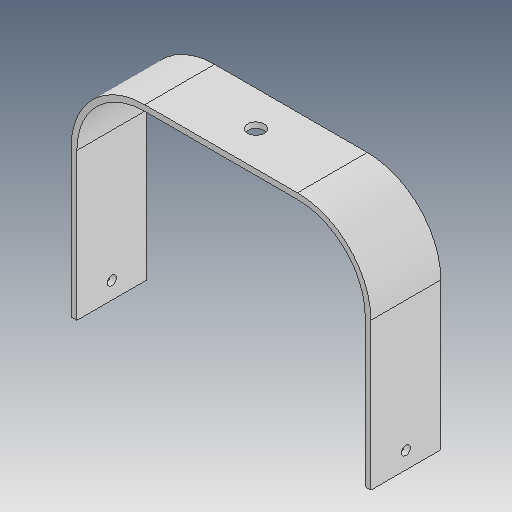
# Autodesk Inventor part: pulley_bracket
Saved by Autodesk Inventor 2025.2 (Build 292293000, 293)
## iProperties
Created: 2025-02-16
Part Number: pulley_bracket
Material: Generic
Document SubType Name: Modeling
Designer: email
Density: 1 g/cm^3
Appearance: Default
Author: email
Autodesk Inventor part; units mm, degrees
ref_plane "YZ Plane" through (0, 0, 0) normal (1, 0, 0) x (0, 1, 0)
ref_plane "XZ Plane" through (0, 0, 0) normal (0, 1, 0) x (-1, 0, 0)
ref_plane "XY Plane" through (0, 0, 0) normal (0, 0, 1) x (1, 0, 0)
sketch "Sketch1" plane through (0, 0, 0) normal (0, 0, 1) x (1, 0, 0)
  line L0 (0, 0) -> (0, 80)
  line L1 (163, 0) -> (163, 80)
  line L2 (0, 0) -> (3.1, 0)
  line L3 (3.1, 0) -> (3.1, 80)
  line L4 (163, 0) -> (159.9, 0)
  line L5 (159.9, 0) -> (159.9, 80)
  arc A0 (40, 116.9) -> (3.1, 80) centre (40, 80) ccw
  arc A1 (159.9, 80) -> (123, 116.9) centre (123, 80) ccw
  line L6 (40, 116.9) -> (123, 116.9)
  arc A2 (40, 120) -> (0, 80) centre (40, 80) ccw
  line L7 (40, 120) -> (123, 120)
  arc A3 (163, 80) -> (123, 120) centre (123, 80) ccw
  dimension "d0" = 163
  dimension "d1" = 80
  dimension "d2" = 3.1
  dimension "d3" = 3.1
  dimension "d4" = 3.1
  dimension "d5" = 120
  constraints: 16 end point, 8 point on circle, 6 tangent, 4 centre point, 4 horizontal, 2 concentric, 2 perpendicular, 2 vertical, 1 collinear, 1 parallel
  measures "d0" distance between parallel lines of L1 L0
  measures "d1" distance of L0.start L0.end
  measures "d2" distance between parallel lines of L0 L3
  measures "d3" distance between parallel lines of L1 L5
  measures "d4" distance between parallel lines of L7 L6
  measures "d5" distance between parallel lines of L7 L2
extrude "Extrusion1" add sketch "Sketch1" along normal blind 38
sketch "Sketch2" plane through (163, 0, 0) normal (1, 0, 0) x (0, 0, -1)
  circle A0 centre (-19, 9.25) radius 2.5
  line L0 (-38, 0) -> (-38, 80) projected
  line L1 (0, 0) -> (-38, 0) projected
  dimension "d8" = 5
  dimension "d9" = 19
  dimension "d10" = 9.25
  constraints: 1 centre point
  measures "d8" diameter of A0
  measures "d9" distance from line of L0 A0.centre
  measures "d10" distance from line of L1 A0.centre
extrude "Extrusion2" cut sketch "Sketch2" against normal through all
sketch "Sketch3" plane through (40, 120, 0) normal (0, 1, 0) x (1, 0, 0)
  circle A0 centre (41.5, -19) radius 4.5
  line L0 (-40, 0) -> (-40, -38) projected
  line L1 (83, 0) -> (0, 0) projected
  point P0 (-40, -19)
  dimension "d13" = 81.5
  dimension "d14" = 19
  dimension "d15" = 9
  constraints: 1 centre point, 1 midpoint
  measures "d13" distance of point (-40, -19) A0.centre
  measures "d14" distance from line of L1 A0.centre
  measures "d15" diameter of A0
extrude "Extrusion3" cut sketch "Sketch3" against normal up to surface (3.1 mm away)
body "Solid1"
